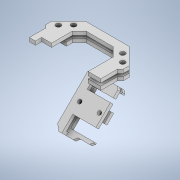
# Autodesk Inventor part: Button Holder
Saved by Autodesk Inventor 2020 (Build 240168000, 168)
## iProperties
Created: 2021-01-14
Part Number: Button Holder
Material: Generic
Document SubType Name: Modeling
Designer: Luke
Density: 1 g/cm^3
Appearance: Default
Author: Luke
Autodesk Inventor part; units mm, degrees
ref_plane "YZ Plane" through (0, 0, 0) normal (1, 0, 0) x (0, 1, 0)
ref_plane "XZ Plane" through (0, 0, 0) normal (0, 1, 0) x (-1, 0, 0)
ref_plane "XY Plane" through (0, 0, 0) normal (0, 0, 1) x (1, 0, 0)
ref_plane "Work Plane1" through (59.9208, 47.0911, 21.911) normal (0, 1, 0) x (-1, 0, 0)
sketch "Sketch1" plane through (59.9208, 47.0911, 21.911) normal (0, 1, 0) x (-1, 0, 0)
  circle A0 centre (-16.808, -43.6345) radius 1.27
  circle A1 centre (12.5729, -47.6345) radius 1.27
  circle A2 centre (16.4459, -43.6345) radius 1.27
  circle A3 centre (-12.808, -47.6345) radius 1.27
  line L0 (10.208, -33.8805) -> (10.208, -44.6601)
  line L1 (10.208, -44.6601) -> (6.6725, -48.1956)
  circle A4 centre (-16.808, -43.6345) radius 1.27 projected
  circle A5 centre (12.5729, -47.6345) radius 1.27 projected
  circle A6 centre (16.4459, -43.6345) radius 1.27 projected
  circle A7 centre (-12.8081, -47.6345) radius 1.27 projected
  line L2 (19.708, -15.6655) -> (-19.708, -15.6655)
  line L3 (0, -15.6655) -> (0, -20.8781)
  line L4 (6.6725, -48.1956) -> (-7.3796, -48.1956)
  line L5 (-19.958, -43.8381) -> (-12.8316, -50.9645)
  line L6 (-12.8316, -50.9645) -> (12.8316, -50.9645)
  line L7 (-19.958, -40.6601) -> (-19.958, -43.8381)
  line L8 (0, -48.1956) -> (0, -46.7038)
  line L9 (19.958, -43.8381) -> (12.8316, -50.9645)
  line L10 (19.958, -40.6601) -> (19.958, -43.8381)
  line L11 (-11.938, -30.6601) -> (-11.938, -43.6372)
  line L12 (-10.5616, -45.0137) -> (-11.938, -43.6372)
  line L13 (-10.5616, -45.0137) -> (-7.3796, -48.1956)
  line L14 (15.2967, -30.6601) -> (18.458, -30.6601)
  line L15 (18.458, -30.6601) -> (18.458, -39.1601)
  line L16 (-18.458, -39.1601) -> (-18.458, -30.6601)
  line L17 (-18.458, -30.6601) -> (-11.938, -30.6601)
  line L18 (10.208, -33.8805) -> (15.2967, -33.8805)
  line L19 (15.2967, -33.8805) -> (15.2967, -30.6601)
  line L20 (-19.958, -40.6601) -> (-18.458, -39.1601)
  line L21 (19.958, -40.6601) -> (18.458, -39.1601)
  point P0 (-19.708, -43.6601)
  point P1 (-6.6725, -48.1956)
  dimension "d14" = 5
  dimension "d15" = 135
  dimension "d18" = 2.54
  constraints: 44 end point, 4 centre point, 4 symmetric about line, 3 vertical, 2 horizontal, 2 point on line, 1 midpoint, 1 perpendicular
  measures "d14" distance of L0.end L1.end
  measures "d15" angle of L0 L1
  measures "d18" diameter of A1
extrude "Extrusion1" add sketch "Sketch1" along normal blind 2
ref_plane "Work Plane2" through (59.9208, 45.8611, 21.911) normal (0, -1, 0) x (1, 0, 0)
sketch "Sketch2" plane through (59.9208, 45.8611, 21.911) normal (0, -1, 0) x (1, 0, 0)
  line L0 (-10.208, -33.8805) -> (-10.208, -44.6601) projected
  line L1 (-10.208, -44.6601) -> (-6.6725, -48.1956) projected
  line L2 (-6.6725, -48.1956) -> (7.3796, -48.1956) projected
  circle A0 centre (16.808, -43.6345) radius 1.27 projected
  circle A1 centre (-12.5729, -47.6345) radius 1.27 projected
  circle A2 centre (-16.4459, -43.6345) radius 1.27 projected
  circle A3 centre (12.808, -47.6345) radius 1.27 projected
  line L3 (19.958, -40.6601) -> (19.958, -43.8381) projected
  line L4 (19.958, -43.8381) -> (12.8316, -50.9645) projected
  line L5 (12.8316, -50.9645) -> (-12.8316, -50.9645) projected
  line L6 (-12.8316, -50.9645) -> (-19.958, -43.8381) projected
  line L7 (-19.958, -43.8381) -> (-19.958, -40.6601) projected
  line L8 (7.3796, -48.1956) -> (11.938, -43.6372) projected
  line L9 (11.938, -43.6372) -> (11.938, -30.6601) projected
  line L10 (11.938, -30.6601) -> (18.458, -30.6601) projected
  line L11 (18.458, -30.6601) -> (18.458, -39.1601) projected
  line L12 (-18.458, -39.1601) -> (-18.458, -30.6601) projected
  line L13 (-18.458, -30.6601) -> (-15.2967, -30.6601) projected
  line L14 (-15.2967, -30.6601) -> (-15.2967, -33.8805) projected
  line L15 (-15.2967, -33.8805) -> (-10.208, -33.8805) projected
  line L16 (18.458, -39.1601) -> (19.958, -40.6601) projected
  line L17 (-19.958, -40.6601) -> (-18.458, -39.1601) projected
  circle A4 centre (-16.4459, -43.6345) radius 1.27 projected
  line L18 (-19.958, -43.8381) -> (-19.958, -40.6601) projected
  line L19 (-19.958, -41.5123) -> (-10.208, -41.5123)
  line L20 (-10.208, -33.8805) -> (-10.208, -44.6601) projected
  point P0 (-59.9208, -21.911)
  constraints: 2 end point, 1 perpendicular, 1 point on line
extrude "Extrusion2" add sketch "Sketch2" along normal blind 2 contours L0 L1 L2 L8 L9 L10 L11 L16 L3 L4 L5 L6 L7 L19
sketch "Sketch4" plane through (79.8789, 45.8611, -18.7491) normal (1, 0, 0) x (0, 0, -1)
  line L0 (0, 1.23) -> (3.178, 1.23) projected
  line L1 (0, 0) -> (-1.5, 0) projected
  line L2 (0, 1.23) -> (0, 0)
  line L3 (-12.1065, -0.085) -> (12.1065, -0.085)
  line L4 (12.1065, -0.085) -> (12.1065, 1.315)
  line L5 (12.1065, 1.315) -> (-12.1065, 1.315)
  line L6 (-12.1065, 1.315) -> (-12.1065, -0.085)
  line L7 (-12.1065, -0.085) -> (12.1065, 1.315) construction
  line L8 (12.1065, -0.085) -> (-12.1065, 1.315) construction
  point P0 (0, 0.615)
  dimension "d73" = 1.4
  constraints: 14 end point, 3 midpoint, 2 parallel, 1 horizontal, 1 perpendicular, 1 vertical
  measures "d73" distance of L4.end L3.end
extrude "Extrusion3" cut sketch "Sketch4" against normal through all
sketch "Sketch5" plane through (59.9208, 43.8611, 21.911) normal (0, -1, 0) x (1, 0, 0)
  line L0 (-19.708, -43.6601) -> (-19.708, -40.6601)
  line L1 (-12.6424, -50.7145) -> (-19.708, -43.6601)
  line L2 (12.728, -50.7145) -> (-12.6424, -50.7145)
  line L3 (19.708, -43.7345) -> (12.728, -50.7145)
  line L4 (-11.3316, -52.4645) -> (11.3316, -52.4645)
  line L5 (19.708, -43.7345) -> (19.708, -40.6601)
  line L6 (-12.8316, -50.9145) -> (12.8316, -50.9145)
  line L7 (12.8316, -50.9645) -> (11.3316, -52.4645)
  line L8 (-19.958, -43.8381) -> (-12.8316, -50.9645) projected
  line L9 (-12.8316, -50.9645) -> (-11.3316, -52.4645)
  line L10 (-12.8316, -50.9645) -> (-10.7103, -50.9645) construction
  line L11 (12.8316, -50.9145) -> (12.8816, -50.9145)
  line L12 (-12.8316, -50.9645) -> (12.8316, -50.9645) projected
  line L13 (12.8316, -50.9645) -> (12.8816, -50.9145)
  line L14 (12.8316, -50.9645) -> (19.958, -43.8381) projected
  line L15 (-12.8316, -50.9145) -> (-12.8816, -50.9145)
  line L16 (-12.8316, -50.9645) -> (-12.8816, -50.9145)
  dimension "d29" = 0.2
  dimension "d62" = 45
  constraints: 28 end point, 3 horizontal, 2 collinear, 1 equal length, 1 point on line
  measures "d29" distance between parallel lines of L2 L6
  measures "d62" angle of L9 L10
extrude "Extrusion4" add sketch "Sketch5" against normal up to surface (5.23 mm away)
ref_plane "Work Plane3" through (59.9523, 18.4601, -23.7213) normal (0, -0.7071068, -0.7071068) x (1, 0, 0)
sketch "Sketch6" plane through (59.9523, 18.4601, -23.7213) normal (0, -0.7071068, -0.7071068) x (1, 0, 0)
  line L0 (-5.715, 11.43) -> (-6.985, 10.16) projected
  line L1 (-6.985, 10.16) -> (-6.985, -10.16) projected
  line L2 (-6.985, -10.16) -> (-5.715, -11.43) projected
  line L3 (-5.715, -11.43) -> (5.715, -11.43) projected
  line L4 (5.715, 11.43) -> (-5.715, 11.43) projected
  circle A0 centre (5.08, 0) radius 0.9525 projected
  circle A1 centre (-5.08, 0) radius 0.9525 projected
  line L5 (6.985, 2.5) -> (-4.985, 2.5)
  line L6 (-4.985, -2.5) -> (6.985, -2.5)
  line L7 (6.985, -2.5) -> (6.985, 2.5)
  line L8 (-4.985, -10.02) -> (6.985, -10.02)
  line L9 (6.965, 10.18) -> (-4.985, 10.18)
  line L10 (-4.985, -10.02) -> (-4.985, -2.5)
  line L11 (-4.985, 2.5) -> (-4.985, 10.18)
  line L12 (7.2325, -10.4075) -> (5.86, -11.78)
  line L13 (5.86, -11.78) -> (-5.86, -11.78)
  line L14 (-5.86, -11.78) -> (-7.335, -10.305)
  line L15 (-7.335, -10.305) -> (-7.335, 10.305)
  line L16 (-7.335, 10.305) -> (-5.86, 11.78)
  line L17 (-5.86, 11.78) -> (5.86, 11.78)
  line L18 (5.86, 11.78) -> (7.2125, 10.4275)
  line L19 (6.985, -10.02) -> (6.985, -10.655)
  line L20 (6.965, 10.18) -> (6.965, 10.675)
  point P0 (-59.9523, 29.8267)
  point P1 (0, 0)
  dimension "d43" = 0.35
  constraints: 32 end point, 2 perpendicular, 2 point on line, 2 vertical, 1 horizontal, 1 parallel, 4 other
  measures "d43" distance between parallel lines of L3 L13
extrude "Extrusion5" add sketch "Sketch6" along normal blind 2
ref_plane "Work Plane5" through (59.9523, 19.3298, -22.8515) normal (0, 0.7071068, 0.7071068) x (-1, 0, 0)
sketch "Sketch7" plane through (59.9523, 19.3298, -22.8515) normal (0, 0.7071068, 0.7071068) x (-1, 0, 0)
  line L0 (4.985, 10.18) -> (-6.965, 10.18) projected
  line L1 (-6.965, 10.18) -> (-6.965, 10.675) projected
  line L2 (-6.965, 10.675) -> (-5.86, 11.78) projected
  line L3 (-5.86, 11.78) -> (5.86, 11.78) projected
  line L4 (5.86, 11.78) -> (7.335, 10.305) projected
  line L5 (7.335, 10.305) -> (7.335, -10.305) projected
  line L6 (7.335, -10.305) -> (5.86, -11.78) projected
  line L7 (5.86, -11.78) -> (-5.86, -11.78) projected
  line L8 (-5.86, -11.78) -> (-6.985, -10.655) projected
  line L9 (-6.985, -10.655) -> (-6.985, -10.02) projected
  line L10 (-6.985, -10.02) -> (4.985, -10.02) projected
  line L11 (4.985, -10.02) -> (4.985, -2.5) projected
  line L12 (4.985, -2.5) -> (-6.985, -2.5) projected
  line L13 (-6.985, -2.5) -> (-6.985, 2.5) projected
  line L14 (-6.985, 2.5) -> (4.985, 2.5) projected
  line L15 (4.985, 2.5) -> (4.985, 10.18) projected
  circle A0 centre (5.08, 0) radius 0.9525 projected
  circle A1 centre (-5.08, 0) radius 0.9525 projected
  line L16 (4.985, -2.5) -> (-6.985, -2.5) projected
  line L17 (4.985, -2.5) -> (-6.985, -2.5)
  line L18 (-6.985, -2.5) -> (-6.985, -5.25)
  line L19 (-6.985, -5.25) -> (4.985, -5.25)
  line L20 (4.985, -5.25) -> (4.985, -2.5)
  line L21 (4.985, 2.5) -> (-6.985, 2.5)
  line L22 (-6.985, 2.5) -> (-6.985, 5.25)
  line L23 (-6.985, 5.25) -> (4.985, 5.25)
  line L24 (4.985, 5.25) -> (4.985, 2.5)
  line L25 (4.985, -10.02) -> (4.985, -2.5) projected
  line L26 (4.985, -10.02) -> (-6.985, -10.02)
  line L27 (-6.985, -10.02) -> (-6.985, -7.29)
  line L28 (-6.985, -7.29) -> (4.985, -7.29)
  line L29 (4.985, -7.29) -> (4.985, -10.02)
  line L30 (4.985, 10.18) -> (4.985, 11.78)
  line L31 (-5.86, 11.78) -> (5.86, 11.78) projected
  point P0 (4.985, 5.25)
  point P1 (4.985, -7.29)
  point P2 (4.985, 11.78)
  dimension "d67" = 11.97
  dimension "d68" = 2.75
  dimension "d69" = 2.75
  constraints: 26 end point, 6 parallel, 4 perpendicular, 3 horizontal, 1 point on line
  measures "d67" distance of L19.end L18.end
  measures "d68" distance of L18.end L17.end
  measures "d69" distance of L21.end L22.end
extrude "Extrusion6" add sketch "Sketch7" along normal blind 2 contours L30 L3 L4 L5 L6 L7 L8 L9 L10 L11 L12 L13 L14 L15 | L15 L14 L22 L23 | L12 L11 L19 L18 | L11 L10 L27 L28
sketch "Sketch8" plane through (66.9373, 16.6923, -21.9535) normal (1, 0, 0) x (0, -0.7071068, -0.7071068)
  line L0 (0, 3.4525) -> (0, 1.5475) projected
  line L1 (0, 2.5) -> (-1.23, 2.5)
  line L2 (-1.23, 1.5475) -> (-1.23, 3.4525) projected
  line L3 (-1.315, 16.5647) -> (0.085, 16.5647)
  line L4 (0.085, 16.5647) -> (0.085, -11.5647)
  line L5 (0.085, -11.5647) -> (-1.315, -11.5647)
  line L6 (-1.315, -11.5647) -> (-1.315, 16.5647)
  line L7 (-1.315, 16.5647) -> (0.085, -11.5647) construction
  line L8 (0.085, 16.5647) -> (-1.315, -11.5647) construction
  point P0 (-3.7202, -27.3267)
  point P1 (-0.615, 2.5)
  dimension "d48" = 1.4
  constraints: 14 end point, 5 midpoint, 2 parallel, 1 horizontal, 1 perpendicular
  measures "d48" distance of L4.end L5.end
extrude "Extrusion7" cut sketch "Sketch8" against normal through all
sketch "Sketch9" plane through (59.9523, 17.0459, -25.1355) normal (0, -0.7071068, -0.7071068) x (-1, 0, 0)
  line L0 (0, -11.78) -> (5.86, -11.78)
  line L1 (5.86, -11.78) -> (7.335, -10.305) projected
  line L2 (7.335, -10.305) -> (7.335, 10.305) projected
  line L3 (7.335, 10.305) -> (5.86, 11.78) projected
  line L4 (5.86, 11.78) -> (0, 11.78)
  line L5 (1.5, 13.28) -> (6.4813, 13.28)
  line L6 (6.4813, 13.28) -> (8.835, 10.9263)
  line L7 (8.835, 10.9263) -> (8.835, -10.9263)
  line L8 (8.835, -10.9263) -> (6.4813, -13.28)
  line L9 (6.4813, -13.28) -> (1.5, -13.28)
  line L10 (-5.86, -11.78) -> (5.86, -11.78) projected
  line L11 (0, 11.78) -> (1.5, 13.28)
  line L12 (0, 11.78) -> (2.1213, 11.78) construction
  line L13 (0, -11.78) -> (1.5, -13.28)
  line L14 (0, -11.78) -> (2.1213, -11.78) construction
  point P0 (4.985, -10.18)
  dimension "d51" = 1.5
  dimension "d65" = 45
  dimension "d66" = 45
  constraints: 22 end point, 2 equal length, 2 horizontal, 2 other
  measures "d51" distance between parallel lines of L4 L5
  measures "d65" angle of L12 L11
  measures "d66" angle of L13 L14
extrude "Extrusion8" add sketch "Sketch9" against normal up to surface (5.23 mm away)
sketch "Sketch10" plane through (59.9523, 20.744, -21.4373) normal (0, 0.7071068, 0.7071068) x (1, 0, 0)
  line L0 (-1.5, -13.28) -> (-4.985, -13.28)
  line L1 (0, -11.78) -> (-1.5, -13.28)
  line L2 (-4.985, -11.78) -> (0, -11.78)
  line L3 (-4.985, -11.78) -> (0, -11.78) projected
  line L4 (-4.985, -11.78) -> (-4.985, -13.28)
  constraints: 8 end point, 1 perpendicular
extrude "Extrusion9" cut sketch "Sketch10" against normal up to surface (3.315 mm away)
body "Solid1"
